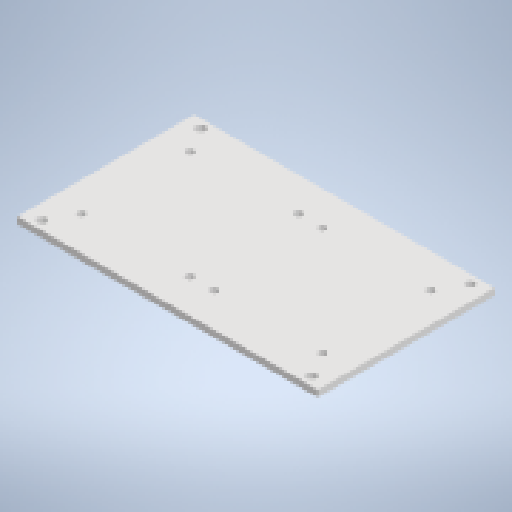
# Autodesk Inventor part: 라즈베리파이 보관소 2층 판
Saved by Autodesk Inventor 2024 (Build 280153000, 153)
## iProperties
Created: 2024-06-03
Part Number: 라즈베리파이 보관소 2층 판
Material: 일반
Document SubType Name: Modeling
Designer: kkamin5
Density: 1 g/cm^3
Appearance: 기본값
Author: kkamin5
Autodesk Inventor part; units mm, degrees
ref_plane "YZ Plane" through (0, 0, 0) normal (1, 0, 0) x (0, 1, 0)
ref_plane "XZ Plane" through (0, 0, 0) normal (0, 1, 0) x (-1, 0, 0)
ref_plane "XY Plane" through (0, 0, 0) normal (0, 0, 1) x (1, 0, 0)
sketch "스케치1" plane through (0, 0, 0) normal (0, 1, 0) x (-1, 0, 0)
  line L0 (-68, 40) -> (68, 40)
  line L1 (68, 40) -> (68, -40)
  line L2 (68, -40) -> (-68, -40)
  line L3 (-68, -40) -> (-68, 40)
  line L4 (-68, 40) -> (68, -40) construction
  line L5 (68, 40) -> (-68, -40) construction
  point P0 (0, 0)
  dimension "d0" = 136
  dimension "d1" = 80
  constraints: 12 end point, 2 midpoint, 2 parallel, 1 horizontal, 1 perpendicular
  measures "d0" distance of L1.end L2.end
  measures "d1" distance of L0.end L1.end
extrude "돌출1" add sketch "스케치1" along normal blind 3
sketch "스케치2" plane through (0, 3, 0) normal (0, 1, 0) x (1, 0, 0)
  circle A0 centre (-54.5, 24.5) radius 1.75
  circle A1 centre (-5.5, 24.5) radius 1.75
  circle A2 centre (5.5, 24.5) radius 1.75
  circle A3 centre (54.5, 24.5) radius 1.75
  circle A4 centre (54.5, -24.5) radius 1.75
  circle A5 centre (5.5, -24.5) radius 1.75
  circle A6 centre (-5.5, -24.5) radius 1.75
  circle A7 centre (-54.5, -24.5) radius 1.75
  circle A8 centre (-61, 36) radius 2
  line L0 (-65, 32) -> (-57, 32)
  line L1 (-57, 32) -> (-57, 40)
  line L2 (-57, 40) -> (-65, 40)
  line L3 (-65, 40) -> (-65, 32)
  line L4 (-65, 32) -> (-57, 40) construction
  line L5 (-57, 32) -> (-65, 40) construction
  line L6 (68, 40) -> (-68, 40) projected
  line L7 (-68, 40) -> (-68, -40) projected
  line L8 (-1.8724, 0) -> (2.8404, 0)
  line L9 (0, 1.8083) -> (0, -2.4649)
  circle A9 centre (61, 36) radius 2
  circle A10 centre (-61, -36) radius 2
  circle A11 centre (61, -36) radius 2
  line L10 (68, -40) -> (68, 40) projected
  line L11 (-68, -40) -> (68, -40) projected
  dimension "d13" = 3.5
  dimension "d14" = 3.5
  dimension "d15" = 3.5
  dimension "d16" = 3.5
  dimension "d17" = 3.5
  dimension "d18" = 3.5
  dimension "d19" = 3.5
  dimension "d20" = 3.5
  dimension "d21" = 4
  dimension "d22" = 8
  dimension "d23" = 4
  dimension "d24" = 8
  dimension "d25" = 7
  dimension "d26" = 13.5
  dimension "d27" = 13.5
  dimension "d28" = 13.5
  dimension "d29" = 13.5
  dimension "d30" = 0
  dimension "d31" = 0
  dimension "d32" = 0
  dimension "d33" = 0
  dimension "d34" = 0
  dimension "d35" = 0
  dimension "d36" = 0
  dimension "d37" = 0
  dimension "d38" = 49
  dimension "d39" = 11
  dimension "d40" = 49
  dimension "d41" = 15.5
  constraints: 16 end point, 12 centre point, 3 symmetric about line, 2 horizontal, 2 midpoint, 2 parallel, 1 perpendicular, 1 vertical, 3 other
  measures "d13" diameter of A0
  measures "d14" diameter of A1
  measures "d15" diameter of A2
  measures "d16" diameter of A3
  measures "d17" diameter of A4
  measures "d18" diameter of A5
  measures "d19" diameter of A6
  measures "d20" diameter of A7
  measures "d21" diameter of A8
  measures "d22" distance of L2.end L1.end
  measures "d23" distance from line of A8.centre L6
  measures "d24" distance of L0.end L1.end
  measures "d25" distance from line of L7 A8.centre
  measures "d26" distance from line of A4.centre L10
  measures "d27" distance from line of L10 A3.centre
  measures "d28" distance from line of L7 A0.centre
  measures "d29" distance from line of L7 A7.centre
  measures "d30" vertical distance of A4.centre A5.centre
  measures "d31" horizontal distance of A5.centre A2.centre
  measures "d32" vertical distance of A3.centre A2.centre
  measures "d33" vertical distance of A2.centre A1.centre
  measures "d34" vertical distance of A1.centre A0.centre
  measures "d35" vertical distance of A7.centre A5.centre
  measures "d36" vertical distance of A7.centre A6.centre
  measures "d37" horizontal distance of A6.centre A1.centre
  measures "d38" distance of A6.centre A1.centre
  measures "d39" distance of A2.centre A1.centre
  measures "d40" distance of A0.centre A1.centre
  measures "d41" distance from line of L11 A4.centre
extrude "돌출2" cut sketch "스케치2" against normal blind 3 contours A0 | A1 | A2 | A3 | A4 | A5 | A6 | A7 | A8 | A9 | A10 | A11
equation "\"d27\" = d26"
equation "\"d28\" = d26"
equation "\"d29\" = d26"
